# Autodesk Inventor part: MMBT2222A
Saved by Autodesk Inventor 2016 SP1 (Build 200210100, 210)
## iProperties
Created: 2015-11-19
Part Number: MMBT2222A
Material: Generic
Document SubType Name: Modeling
Designer: PhillipD
Density: 1 g/cm^3
Appearance: SOT23-3, MMBT2222A
Author: PhillipD
Autodesk Inventor part; units mm, degrees
ref_plane "YZ Plane" through (0, 0, 0) normal (1, 0, 0) x (0, 1, 0)
ref_plane "XZ Plane" through (0, 0, 0) normal (0, 1, 0) x (-1, 0, 0)
ref_plane "XY Plane" through (0, 0, 0) normal (0, 0, 1) x (1, 0, 0)
sketch "SOT23-3, MMBT2222A_30" plane through (0, 0, 0) normal (0, 0, 1) x (1, 0, 0)
  line L0 (-1.4224, 0.7366) -> (1.4986, 0.7366)
  line L1 (1.4986, 0.7366) -> (1.4986, -0.7366)
  line L2 (1.4986, -0.7366) -> (-1.4224, -0.7366)
  line L3 (-1.4224, -0.7366) -> (-1.4224, 0.7366)
  constraints: 8 end point
extrude "Extrusion1" add sketch "SOT23-3, MMBT2222A_30" along normal blind 1
body "Solid1"
